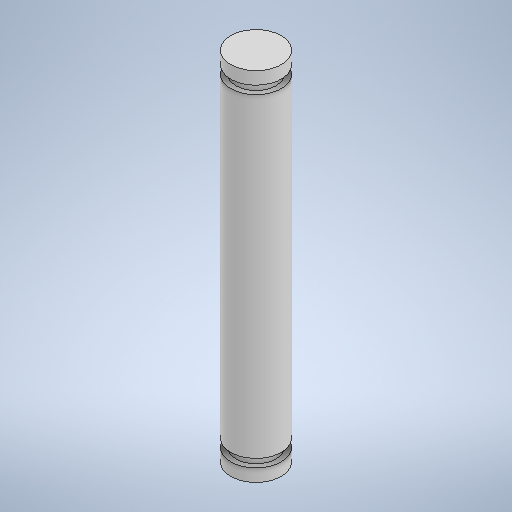
# Autodesk Inventor part: Kipphebelachse
Saved by Autodesk Inventor 2025 (Build 290162010, 162A)
## iProperties
Created: 2024-04-30
Part Number: Kipphebelachse
Material: Generisch
Document SubType Name: Modeling
Designer: ffogue
Density: 1 g/cm^3
Appearance: Vorgabe
Author: ffogue
Autodesk Inventor part; units mm, degrees
ref_plane "YZ Plane" through (0, 0, 0) normal (1, 0, 0) x (0, 1, 0)
ref_plane "XZ Plane" through (0, 0, 0) normal (0, 1, 0) x (-1, 0, 0)
ref_plane "XY Plane" through (0, 0, 0) normal (0, 0, 1) x (1, 0, 0)
sketch "Skizze1" plane through (0, 0, 0) normal (0, 1, 0) x (-1, 0, 0)
  line L0 (0, 0) -> (2, 0)
  line L1 (2, 0) -> (2, -1)
  line L2 (2, -1) -> (1.6, -1)
  line L3 (1.6, -1) -> (1.6, -1.65)
  line L4 (1.6, -1.65) -> (2, -1.65)
  line L5 (2, -1.65) -> (2, -26.65)
  line L6 (2, -26.65) -> (1.6, -26.65)
  line L7 (1.6, -26.65) -> (1.6, -27.3)
  line L8 (1.6, -27.3) -> (2, -27.3)
  line L9 (2, -27.3) -> (2, -28.3)
  line L10 (2, -28.3) -> (0, -28.3)
  line L11 (0, 0) -> (0, -28.3)
  dimension "d0" = 2
  dimension "d1" = 1
  dimension "d2" = 0.65
  dimension "d3" = 0.65
  dimension "d5" = 1
  dimension "d6" = 4
  dimension "d7" = 3.2
  dimension "d9" = 25
  constraints: 24 end point, 6 perpendicular, 4 point on line, 2 vertical, 1 collinear, 1 horizontal, 1 parallel
  measures "d0" distance of L0.start L0.end
  measures "d1" distance of L0.end L1.end
  measures "d2" distance of L2.end L3.end
  measures "d3" distance of L6.end L7.end
  measures "d5" distance between parallel lines of L10 L8
  measures "d6" diameter of L5 L11
  measures "d7" diameter of L7 L11
  measures "d9" distance of L4.end L5.end
revolve "Umdrehung1" add sketch "Skizze1" angle 360 about axis through (0, 0, 0) along (0, 0, -1)
